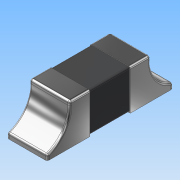
# Autodesk Inventor part: BLM18PG471SN1D Ferrite Bead
Saved by Autodesk Inventor 2016 (Build 200138000, 138)
## iProperties
Created: 2019-08-18
Part Number: BLM18PG471SN1D Ferrite Bead
Material: Laminate, Ivory, Matte
Document SubType Name: Modeling
Designer: Orest
Mass: 0.0016283 g
Surface Area: 0.0772739 cm^2
Volume: 0.00117993 cm^3
Density: 1.38 g/cm^3
Appearance: Smooth - Black (BGA)
Author: Orest
Autodesk Inventor part; units mm, degrees
ref_plane "YZ Plane" through (0, 0, 0) normal (1, 0, 0) x (0, 1, 0)
ref_plane "XZ Plane" through (0, 0, 0) normal (0, 1, 0) x (-1, 0, 0)
ref_plane "XY Plane" through (0, 0, 0) normal (0, 0, 1) x (1, 0, 0)
sketch "Sketch10" plane through (0, 0, 0) normal (0, 0, 1) x (1, 0, 0)
  line L0 (-0.4, 0.3875) -> (0.4, 0.3875)
  line L1 (0.4, 0.3875) -> (0.4, -0.3875)
  line L2 (0.4, -0.3875) -> (-0.4, -0.3875)
  line L3 (-0.4, -0.3875) -> (-0.4, 0.3875)
  point P0 (0, 0)
  point P1 (-0.4, 0)
  point P2 (0, 0.3875)
  dimension "d7" = 0.8
  dimension "d8" = 0.775
  constraints: 8 end point, 2 midpoint, 2 parallel, 1 horizontal, 1 horizontal alignment, 1 perpendicular, 1 vertical alignment
  measures "d7" distance of L1.end L2.end
  measures "d8" distance of L0.end L1.end
extrude "Extrusion4" add sketch "Sketch10" along normal mid plane 0.775
sketch "Sketch11" plane through (0.4, -0.3875, 0.3875) normal (1, 0, 0) x (0, 0, -1)
  line L0 (0, 0.775) -> (0.775, 0.775) construction
  line L1 (0, 0) -> (0, 0.775) construction
  line L2 (0, 0) -> (0.775, 0) construction
  line L3 (0.775, 0.775) -> (0.775, 0) construction
  line L4 (0.7875, 0.7875) -> (-0.0125, 0.7875)
  line L5 (-0.0125, 0.7875) -> (-0.0125, -0.0125)
  line L6 (-0.0125, -0.0125) -> (0.7875, -0.0125)
  line L7 (0.7875, -0.0125) -> (0.7875, 0.7875)
  line L8 (-0.0125, -0.0125) -> (0.7875, -0.0125)
  line L9 (0.7875, -0.0125) -> (0.7875, 0.0875)
  line L10 (0.7875, 0.0875) -> (-0.0125, 0.0875)
  line L11 (-0.0125, 0.0875) -> (-0.0125, -0.0125)
  point P0 (0.3875, 0.3875)
  dimension "d11" = 0.8
  dimension "d14" = 0.1
  constraints: 16 end point, 2 parallel, 1 horizontal, 1 perpendicular, 1 point on line, 3 other
  measures "d11" distance of L4.start L4.end
  measures "d14" distance between parallel lines of L6 L10
extrude "Extrusion5" add sketch "Sketch11" along normal blind 0.4
extrude "Extrusion6" add sketch "Sketch11" along normal blind 0.85 contours L7 L6 L5 L10
fillet "Fillet1" radius 0.65 1 edges at (0.8, -0.3, 0)
fillet "Fillet2" radius 0.0425 10 edges at (0.6, 0.4, -0.4) (0.6, 0.4, 0.4) (0.8, 0.3592, 0.4) (0.9244, -0.064, 0.4) (0.8, 0.3592, -0.4) (0.9244, -0.064, -0.4) (1.25, -0.35, -0.4) (1.25, -0.3, 0) (0.8, 0.4, 0) (1.25, -0.35, 0.4)
mirror "Mirror1" about plane through (0, 0, 0) normal (1, 0, 0) of "Extrusion5", "Fillet1", "Fillet2", "Extrusion6"
fillet "Fillet3" radius 0.03 4 edges at (0, 0.3875, -0.3875) (0, 0.3875, 0.3875) (0, -0.3875, -0.3875) (0, -0.3875, 0.3875)
equation "\"d9\" = d8"
body "Solid4"
